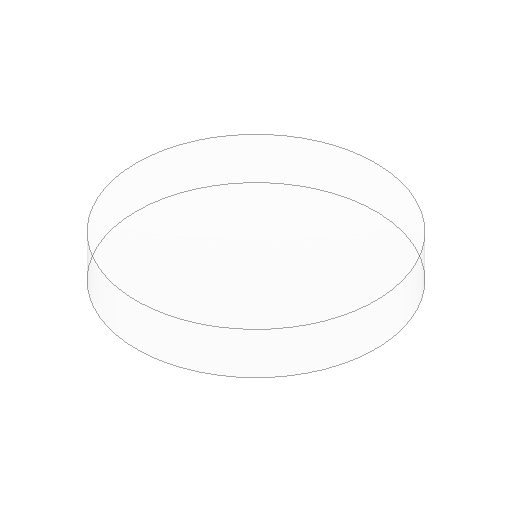
# Autodesk Inventor part: 00_Lens_neg_50mm_India
Saved by Autodesk Inventor 2022 (Build 260153000, 153)
## iProperties
Created: 2022-07-29
Part Number: 00_Lens_neg_50mm_India
Material: Generisch
Document SubType Name: Modeling
Designer: UC2
Density: 1 g/cm^3
Appearance: Polycarbonat - klar
Mass: 6.77723 g
Surface Area: 34.0937 cm^2
Volume: 6.77723 cm^3
Catalog Web Link: http://www.shincoscientificapparatus.com/lenses-spherical-unmounted-4406354.html
Description: Need a revision
Author: UC2
Autodesk Inventor part; units mm, degrees
ref_plane "YZ Plane" through (0, 0, 0) normal (1, 0, 0) x (0, 1, 0)
ref_plane "XZ Plane" through (0, 0, 0) normal (0, 1, 0) x (-1, 0, 0)
ref_plane "XY Plane" through (0, 0, 0) normal (0, 0, 1) x (1, 0, 0)
sketch "Skizze1" plane through (0, 0, 0) normal (0, 0, 1) x (1, 0, 0)
  line L0 (20, -3.5) -> (-20, -3.5)
  line L1 (-20, -3.5) -> (-20, 3.5)
  line L2 (-20, 3.5) -> (20, 3.5)
  line L3 (20, 3.5) -> (20, -3.5)
  line L4 (20, -3.5) -> (-20, 3.5) construction
  line L5 (-20, -3.5) -> (20, 3.5) construction
  arc A0 (-20, 3.5) -> (20, 3.5) centre (0, 147.2231) ccw
  arc A1 (20, -3.5) -> (-20, -3.5) centre (0, -112.3854) ccw
  line L6 (0, 2.1151) -> (0, -1.6784)
  point P0 (0, 0)
  dimension "d0" = 40
  dimension "d1" = 7
  constraints: 14 end point, 6 point on circle, 2 centre point, 2 midpoint, 2 parallel, 1 horizontal, 1 perpendicular
  measures "d0" distance of L1.end L2.end
  measures "d1" distance of L0.end L1.end
revolve "Umdrehung1" add sketch "Skizze1" angle 360 about axis through (0, 2.1151, 0) along (0, -1, 0) contours L1 A0 L6 A1
